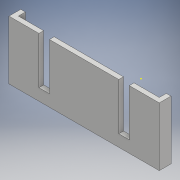
# Autodesk Inventor part: IR Lock Mount
Saved by Autodesk Inventor 2018 (Build 220112000, 112)
## iProperties
Created: 2017-07-06
Part Number: IR Lock Mount
Material: Generic
Document SubType Name: Modeling
Designer: klyu
Density: 1 g/cm^3
Appearance: Default
Author: klyu
Autodesk Inventor part; units mm, degrees
ref_plane "YZ Plane" through (0, 0, 0) normal (1, 0, 0) x (0, 1, 0)
ref_plane "XZ Plane" through (0, 0, 0) normal (0, 1, 0) x (-1, 0, 0)
ref_plane "XY Plane" through (0, 0, 0) normal (0, 0, 1) x (1, 0, 0)
sketch "Sketch1" plane through (0, 0, 0) normal (0, 1, 0) x (-1, 0, 0)
  line L0 (0, 0) -> (4.5, 0)
  line L1 (4.5, 0) -> (4.5, -20)
  line L2 (4.5, -20) -> (0, -20)
  line L3 (0, -20) -> (0, 0)
  line L4 (34, 0) -> (38.5, 0)
  line L5 (38.5, 0) -> (38.5, -20)
  line L6 (38.5, -20) -> (34, -20)
  line L7 (34, -20) -> (34, 0)
  line L8 (51.25, 0) -> (-12.75, 0)
  line L9 (-12.75, 0) -> (-12.75, -25)
  line L10 (-12.75, -25) -> (51.25, -25)
  line L11 (51.25, -25) -> (51.25, 0)
  line L12 (19.25, 0) -> (19.25, -42)
  dimension "d0" = 4.5
  dimension "d1" = 20
  dimension "d2" = 4.5
  dimension "d3" = 20
  dimension "d4" = 38.5
  dimension "d5" = 25
  dimension "d6" = 64
  dimension "d7" = 14.75
  dimension "d8" = 32
  constraints: 26 end point, 6 parallel, 3 horizontal, 3 perpendicular, 2 collinear, 1 midpoint, 1 vertical
  measures "d0" distance between parallel lines of L1 L3
  measures "d1" distance between parallel lines of L2 L0
  measures "d2" distance between parallel lines of L5 L7
  measures "d3" distance between parallel lines of L6 L4
  measures "d4" distance between parallel lines of L3 L5
  measures "d5" distance between parallel lines of L10 L8
  measures "d6" distance between parallel lines of L9 L11
  measures "d7" distance between parallel lines of L12 L7
  measures "d8" distance between parallel lines of L12 L11
extrude "Extrusion1" add sketch "Sketch1" along normal blind 2 contours L3 L2 L1 L8 L12 L10 L9 | L8 L7 L6 L5 L11 L10 L12
sketch "Sketch2" plane through (0, 2, 0) normal (0, 1, 0) x (1, 0, 0)
  line L0 (0, 0) -> (12.75, 0) projected
  line L1 (12.75, 0) -> (10.75, 0)
  line L2 (10.75, 0) -> (10.75, 25)
  line L3 (10.75, 25) -> (12.75, 25)
  line L4 (12.75, 25) -> (12.75, 0)
  line L5 (12.75, 25) -> (-51.25, 25) projected
  line L6 (-49.25, 0) -> (-51.25, 0)
  line L7 (-51.25, 0) -> (-51.25, 25)
  line L8 (-51.25, 25) -> (-49.25, 25)
  line L9 (-49.25, 25) -> (-49.25, 0)
  line L10 (-51.25, 25) -> (-51.25, 0) projected
  line L11 (-51.25, 0) -> (-38.5, 0) projected
  point P0 (13.75, 26)
  dimension "d11" = 2
  dimension "d12" = 2
  constraints: 14 end point, 4 collinear, 3 parallel, 2 horizontal, 2 perpendicular, 1 vertical, 3 other
  measures "d11" distance between parallel lines of L4 L2
extrude "Extrusion2" add sketch "Sketch2" along normal blind 3
sketch "Sketch3" plane through (0, 5, 0) normal (0, 1, 0) x (1, 0, 0)
  point P0 (0, 0)
body "Solid1"
